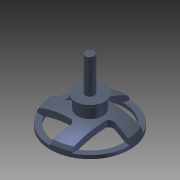
# Autodesk Inventor part: cover
Saved by Autodesk Inventor 2012 (Build 160160000, 160)
## iProperties
Created: 2014-07-09
Part Number: cover
Material: Default
Document SubType Name: Modeling
Designer: Anon
Density: 1 g/cm^3
Author: Anon
Autodesk Inventor part; units mm, degrees
ref_plane "YZ Plane" through (0, 0, 0) normal (1, 0, 0) x (0, 1, 0)
sketch "Sketch4" plane through (0, 0, 0) normal (0, 1, 0) x (-1, 0, 0)
  line L0 (0, 0) -> (0, 7)
  line L1 (0, 0) -> (-17.25, 0)
  line L2 (-17.25, 0) -> (-17.25, 3.2)
  arc A0 (0, 7) -> (-17.25, 3.2) centre (-1.3391, -27.9744) ccw
  line L3 (0, -35.1905) -> (0, 15.3222) projected
  dimension "d25" = 7
  dimension "d26" = 17.25
  dimension "d27" = 3.2
  dimension "d28" = 35
  constraints: 6 end point, 2 perpendicular, 2 point on circle, 1 centre point, 1 vertical
  measures "d25" distance of L0.start L0.end
  measures "d26" distance of L0.start L1.end
  measures "d27" distance of L1.end L2.end
  measures "d28" radius of A0
revolve "Revolution1" add sketch "Sketch4" angle 360 about axis through (0, 0, -10) along (0, 0, 1)
ref_plane "Work Plane2" through (0, 0, 1.5) normal (0, 0, 1) x (1, 0, 0)
sketch "Sketch2" plane through (0, 0, 1.5) normal (0, 0, 1) x (1, 0, 0)
  circle A0 centre (0, 0) radius 14.65 projected
  circle A1 centre (0, 0) radius 17.25 projected
  line L0 (-21.39, 7) -> (20.1238, 7) construction
  line L1 (-21.9779, 1.4) -> (22.4301, 1.4) construction
  line L2 (7.6, 10.9663) -> (7.6, -9.9262) construction
  line L3 (17.25, 0) -> (7.6, 1.4)
  line L4 (7.6, 1.4) -> (7.6, -15.4856)
  arc A2 (7.6, -15.4856) -> (17.25, 0) centre (0, 0) ccw
  line L5 (0, 17.25) -> (-1.4, 7.6)
  line L6 (-1.4, 7.6) -> (15.4856, 7.6)
  arc A3 (15.4856, 7.6) -> (0, 17.25) centre (0, 0) ccw
  line L7 (-17.25, 0) -> (-7.6, -1.4)
  line L8 (-7.6, -1.4) -> (-7.6, 15.4856)
  arc A4 (-7.6, 15.4856) -> (-17.25, 0) centre (0, 0) ccw
  line L9 (0, -17.25) -> (1.4, -7.6)
  line L10 (1.4, -7.6) -> (-15.4856, -7.6)
  arc A5 (-15.4856, -7.6) -> (0, -17.25) centre (0, 0) ccw
  point P0 (9.9262, 7.6)
  point P1 (-7.6, 9.9262)
  point P2 (-9.9262, -7.6)
  dimension "d4" = 7
  dimension "d5" = 5.6
  dimension "d6" = 7.6
  dimension "d16" = 360
  constraints: 22 end point, 10 point on circle, 4 centre point, 3 point on line, 1 coincident, 1 horizontal, 1 parallel, 1 perpendicular, 33 other
  measures "d4" distance from line of A0.centre L0
  measures "d5" distance between parallel lines of L1 L0
  measures "d6" distance from line of L2 A0.centre
sketch "Sketch5" plane through (0, 0, 0) normal (0, 0, -1) x (-1, 0, 0)
  circle A0 centre (0, 0) radius 17.25 projected
  circle A1 centre (0, 0) radius 14.75
  dimension "d30" = 2.5
  constraints: 1 centre point, 1 coincident
  measures "d30" radial gap between concentric circles of A0 A1
extrude "Extrusion3" cut sketch "Sketch5" against normal blind 1.5 contours A1
extrude "Extrusion4" cut sketch "Sketch2" along normal through all contours A0 L4 L3 | A0 L3 A1 L4 | L6 L5 A0 | A0 L5 A1 L6 | L9 A1 L10 A0 | A0 L10 L9 | L8 L7 A0 | A0 L7 A1 L8
chamfer "Chamfer1" distance 1 angle 45 4 edges at (16.8031, 3.9011, 3.2) (-3.9011, 16.8031, 3.2) (-16.8031, -3.9011, 3.2) (3.9011, -16.8031, 3.2)
fillet "Fillet1" radius 2 4 edges at (-1.4, 7.6, 3.9688) (7.6, 1.4, 3.9688) (-7.6, -1.4, 3.9688) (1.4, -7.6, 3.9688)
ref_plane "Work Plane3" through (0, 0, 6.5) normal (0, 0, 1) x (1, 0, 0)
sketch "Sketch6" plane through (0, 0, 6.5) normal (0, 0, 1) x (1, 0, 0)
  circle A0 centre (0, 0) radius 5.5
  dimension "d40" = 11
  constraints: 1 centre point, 1 coincident
  measures "d40" diameter of A0
extrude "Extrusion5" add sketch "Sketch6" along normal blind 4.5
sketch "Sketch7" plane through (0, 0, 11) normal (0, 0, 1) x (1, 0, 0)
  circle A0 centre (0, 0) radius 5.5 projected
  circle A1 centre (0, 0) radius 6.5
  dimension "d43" = 13
  constraints: 1 centre point, 1 coincident
  measures "d43" diameter of A1
extrude "Extrusion6" add sketch "Sketch7" along normal blind 1.75 contours A0 | A1
chamfer "Chamfer2" distance 1 angle 45 1 edges at (-6.5, 0, 11)
sketch "Sketch8" plane through (0, 0, 12.75) normal (0, 0, 1) x (1, 0, 0)
  circle A0 centre (0, 0) radius 6.5 projected
  circle A1 centre (0, 0) radius 1.975
  dimension "d49" = 3.95
  constraints: 1 centre point, 1 coincident
  measures "d49" diameter of A1
extrude "Extrusion7" add sketch "Sketch8" along normal blind 15 contours A1
fillet "Fillet2" radius 0.2 1 edges at (-1.975, 0, 27.75)
sketch "Sketch11" plane through (0, 0, 0) normal (0, 1, 0) x (-1, 0, 0)
  line L0 (0, 1.5) -> (14.6953, 1.5)
  line L1 (0, 1.5) -> (0, 5)
  arc A0 (14.6953, 1.5) -> (0, 5) centre (-3.6349, -42.8622) ccw
  line L2 (0, -58.9387) -> (0, 42.1981) projected
  point P0 (0, 0)
  dimension "d56" = 3.5
  dimension "d57" = 48
  dimension "d58" = 1.5
  constraints: 4 end point, 2 point on circle, 1 centre point, 1 horizontal, 1 perpendicular
  measures "d56" distance of L0.start L1.end
  measures "d57" radius of A0
  measures "d58" distance of L0.start point (0, 0)
revolve "Revolution2" cut sketch "Sketch11" angle 360 about axis through (0, 0, -10) along (0, 0, 1)
body "Solid1"
